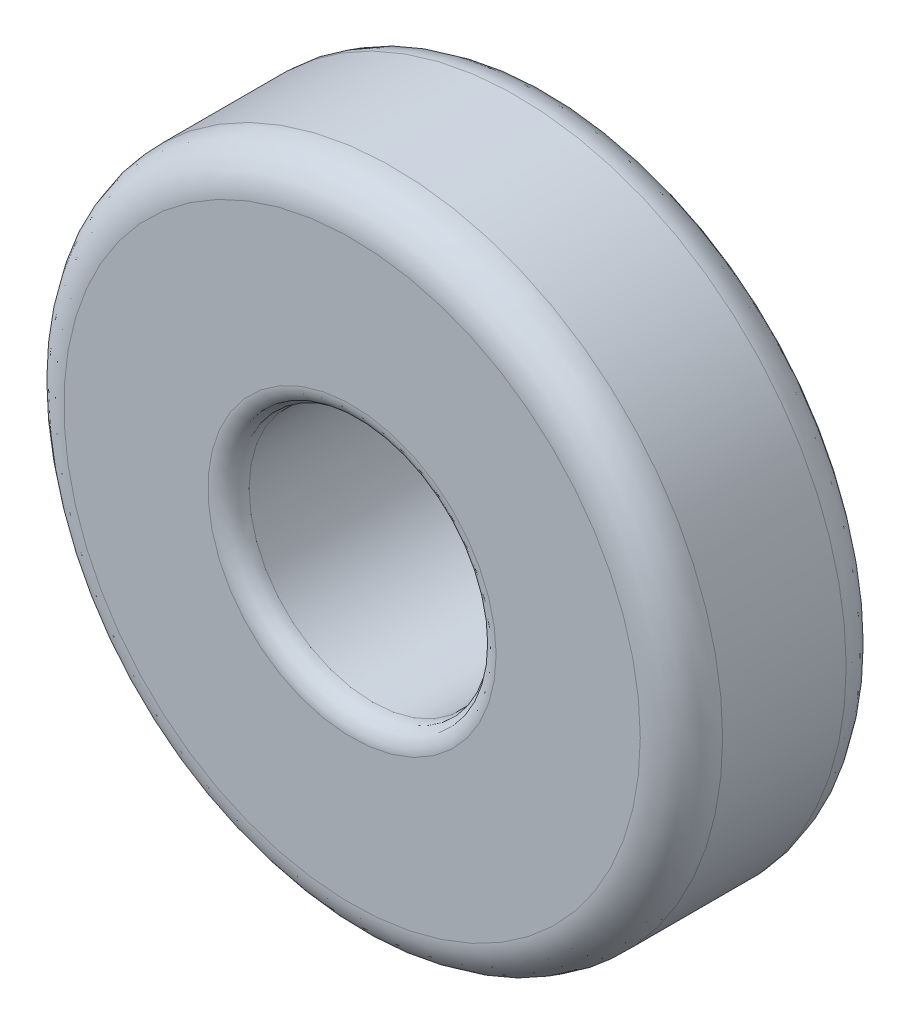
# Autodesk Inventor part: 6201RS
Saved by Autodesk Inventor 2017 SP1 (Build 210196100, 196)
## iProperties
Created: 2017-06-04
Part Number: 6201RS
Material: Steel, Carbon
Catalog Web Link: https://www.amazon.com/uxcell-6201RS-Shielded-Groove-Bearing/dp/B00E0ERMH6/ref=sr_1_1?ie=UTF8&qid=1496593964&sr=8-1&keywords=bearing+12mm
Document SubType Name: Modeling
Designer: Zach
Density: 7.85 g/cm^3
Appearance: Semi-Polished
Author: Zach
Autodesk Inventor part; units mm, degrees
ref_plane "YZ Plane" through (0, 0, 0) normal (1, 0, 0) x (0, 1, 0)
ref_plane "XZ Plane" through (0, 0, 0) normal (0, 1, 0) x (-1, 0, 0)
ref_plane "XY Plane" through (0, 0, 0) normal (0, 0, 1) x (1, 0, 0)
sketch "Sketch1" plane through (0, 0, 0) normal (0, 0, 1) x (1, 0, 0)
  circle A0 centre (0, 0) radius 16
  circle A1 centre (0, 0) radius 6
  dimension "d0" = 32
  dimension "d1" = 12
  constraints: 2 centre point, 2 coincident
  measures "d0" diameter of A0
  measures "d1" diameter of A1
extrude "Extrusion1" add sketch "Sketch1" along normal blind 10
fillet "Fillet1" radius 2 2 edges at (-16, 0, 10) (-16, 0, 0)
fillet "Fillet2" radius 1 2 edges at (-6, 0, 10) (-6, 0, 0)
body "Solid1"
